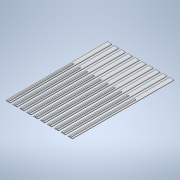
# Autodesk Inventor part: structure4
Saved by Autodesk Inventor 2022 (Build 260153000, 153)
## iProperties
Created: 2022-04-07
Part Number: structure4
Material: Generic
Document SubType Name: Modeling
Designer: ten26
Density: 1 g/cm^3
Appearance: Default
Author: ten26
Autodesk Inventor part; units mm, degrees
ref_plane "YZ Plane" through (0, 0, 0) normal (1, 0, 0) x (0, 1, 0)
ref_plane "XZ Plane" through (0, 0, 0) normal (0, 1, 0) x (-1, 0, 0)
ref_plane "XY Plane" through (0, 0, 0) normal (0, 0, 1) x (1, 0, 0)
sketch "Sketch1" plane through (0, 0, 0) normal (0, 1, 0) x (-1, 0, 0)
  line L0 (2.65, -62.5) -> (-2.65, -62.5)
  line L1 (-2.65, -62.5) -> (-2.65, 62.5)
  line L2 (-2.65, 62.5) -> (2.65, 62.5)
  line L3 (2.65, 62.5) -> (2.65, -62.5)
  line L4 (2.65, -62.5) -> (-2.65, 62.5) construction
  line L5 (-2.65, -62.5) -> (2.65, 62.5) construction
  point P0 (0, 0)
  dimension "d0" = 5.3
  dimension "d1" = 125
  constraints: 12 end point, 2 midpoint, 2 parallel, 1 horizontal, 1 perpendicular
  measures "d0" distance of L1.end L2.end
  measures "d1" distance of L0.end L1.end
extrude "Extrusion1" add sketch "Sketch1" along normal blind 0.5
sketch "Sketch2" plane through (0, 0.5, 0) normal (0, 1, 0) x (1, 0, 0)
  line L0 (-2.65, -62.5) -> (2.65, -62.5) projected
  line L1 (0.65, -62.5) -> (-0.65, -62.5)
  line L2 (-0.65, -62.5) -> (-0.65, 17.5)
  line L3 (-0.65, 17.5) -> (0.65, 17.5)
  line L4 (0.65, 17.5) -> (0.65, -62.5)
  line L5 (-2.65, 62.5) -> (-2.65, -62.5) projected
  point P0 (0, 0)
  dimension "d4" = 1.3
  dimension "d5" = 80
  dimension "d6" = 5.3
  dimension "d7" = 1.3
  dimension "d8" = 2
  constraints: 8 end point, 2 parallel, 1 horizontal, 1 perpendicular, 1 point on line
  measures "d4" distance of L2.end L3.end
  measures "d5" distance from line of L3 L1.start
  measures "d6" distance of L0.start L0.end
  measures "d7" distance between parallel lines of L4 L2
  measures "d8" distance between parallel lines of L2 L5
extrude "Extrusion2" add sketch "Sketch2" along normal blind 0.7
pattern_linear "Rectangular Pattern1" count 10 spacing 8.5 along (1, 0, 0) of "Extrusion1", "Extrusion2"
equation "\"d8\" = 0.5 * d6 - 0.5 * d7"
body "Solid1"
